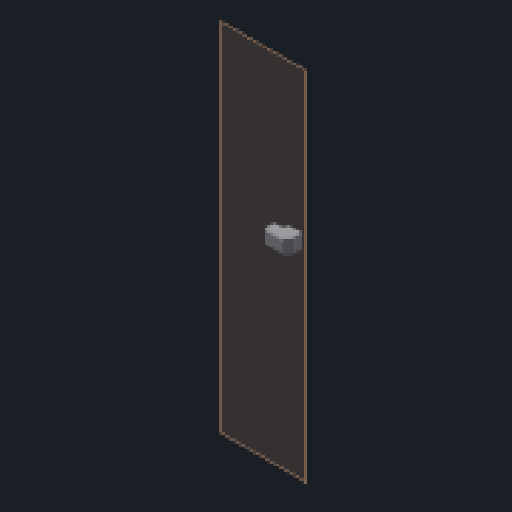
# Autodesk Inventor part: soporte_sensor_puerta
Saved by Autodesk Inventor 2024.3 (Build 283343000, 343)
## iProperties
Created: 2024-08-14
Part Number: soporte_sensor_puerta
Material: Generic
Document SubType Name: Modeling
Designer: Niler
Density: 1 g/cm^3
Appearance: Default
Author: Niler
Autodesk Inventor part; units mm, degrees
ref_plane "YZ Plane" through (0, 0, 0) normal (1, 0, 0) x (0, 1, 0)
ref_plane "XZ Plane" through (0, 0, 0) normal (0, 1, 0) x (-1, 0, 0)
ref_plane "XY Plane" through (0, 0, 0) normal (0, 0, 1) x (1, 0, 0)
ref_plane "Work Plane1" through (0, 0, 0) normal (0, 0, 1) x (1, 0, 0)
sketch "Sketch1" plane through (0, 0, 0) normal (0, 0, 1) x (1, 0, 0)
  line L0 (76.5873, -14.7582) -> (76.5873, 185.2418) projected
  line L1 (76.5873, 107.7418) -> (116.5873, 107.7418)
  line L2 (116.5873, 107.7418) -> (116.5873, 62.7418)
  line L3 (116.5873, 62.7418) -> (76.5873, 62.7418)
  line L4 (76.5873, 62.7418) -> (76.5873, 107.7418)
  point P0 (0, 0)
  point P1 (116.5873, 85.2418)
  point P2 (76.5873, 85.2418)
  point P3 (76.5873, 62.7418)
  dimension "d0" = 45
  dimension "d1" = 40
  constraints: 8 end point, 2 midpoint, 2 parallel, 1 horizontal, 1 horizontal alignment, 1 perpendicular, 1 point on line
  measures "d0" distance of L1.end L2.end
  measures "d1" distance of L2.end L3.end
extrude "Extrusion1" add sketch "Sketch1" along normal blind 45
sketch "Sketch2" plane through (76.5873, 62.7418, 0) normal (-1, 0, 0) x (0, 0, 1)
  line L0 (0, 45) -> (0, 0) projected
  line L1 (0, 0) -> (45, 0) projected
  line L2 (45, 45) -> (45, 0) projected
  line L3 (0, 45) -> (45, 45) projected
  circle A0 centre (29.5, 22.5) radius 9
  point P0 (0, -62.7418)
  point P1 (45, 22.5)
  dimension "d4" = 18
  dimension "d5" = 15.5
  constraints: 1 centre point, 1 horizontal alignment, 1 midpoint
  measures "d4" diameter of A0
  measures "d5" distance from line of A0.centre L2
extrude "Extrusion2" cut sketch "Sketch2" against normal through all contours A0
sketch "Sketch3" plane through (76.5873, 107.7418, 0) normal (0, 1, 0) x (1, 0, 0)
  line L0 (-8, -15) -> (0, -7) projected
  line L1 (-145.0873, -15) -> (-8, -15) projected
  line L2 (-30, -15) -> (-30, -45)
  line L3 (40, 0) -> (0, 0) projected
  line L4 (0, 0) -> (0, -45) projected
  line L5 (40, -45) -> (0, -45) projected
  line L6 (40, 0) -> (40, -45) projected
  line L7 (0, -45) -> (-30, -45)
  point P0 (-76.5873, 0)
  point P1 (0, -7)
  dimension "d8" = 30
  constraints: 5 end point, 1 perpendicular, 1 point on line, 1 vertical
  measures "d8" distance of L4.end L2.end
extrude "Extrusion3" add sketch "Sketch3" against normal up to surface (45 mm away) contours L0 L4 L7 L2 L1
sketch "Sketch4" plane through (46.5873, 107.7418, 15) normal (-1, 0, 0) x (0, 0, 1)
  circle A0 centre (14.5, -22.5) radius 9 projected
  point P0 (-15, -107.7418)
extrude "Extrusion4" cut sketch "Sketch4" against normal through all
chamfer "Chamfer1" distance 15 angle 45 1 edges at (116.5873, 85.2418, 45)
sketch "Sketch5" plane through (101.5873, 62.7418, 45) normal (0.7071068, 0, 0.7071068) x (0.7071068, 0, -0.7071068)
  line L0 (21.2132, 45) -> (0, 45) projected
  line L1 (0, 45) -> (0, 0) projected
  line L2 (0, 0) -> (21.2132, 0) projected
  line L3 (21.2132, 0) -> (21.2132, 13.5139) projected
  ellipse E0 centre (21.9203, 22.5) end of major axis (9.1924, 22.5) minor radius 9 (21.2132, 31.4861) -> (21.2132, 13.5139) ccw projected
  line L4 (21.2132, 31.4861) -> (21.2132, 45) projected
  ellipse E1 centre (21.9203, 22.5) end of major axis (9.1924, 22.5) minor radius 9 (21.2132, 31.4861) -> (21.2132, 13.5139) ccw projected
  line L5 (21.2132, 31.4861) -> (21.2132, 13.5139)
  point P0 (-40.0133, -62.7418)
  constraints: 2 end point, 1 vertical, 2 other
extrude "Extrusion5" add sketch "Sketch5" against normal blind 2
sketch "Sketch6" plane through (116.5873, 62.7418, 0) normal (1, 0, 0) x (0, 0, -1)
  line L0 (-30, 31.4861) -> (-30, 45) projected
  arc A0 (-30, 13.5139) -> (-30, 31.4861) centre (-29.5, 22.5) ccw projected
  line L1 (-30, 0) -> (-30, 13.5139) projected
  line L2 (0, 0) -> (-30, 0) projected
  line L3 (0, 0) -> (0, 45) projected
  line L4 (0, 45) -> (-30, 45) projected
  line L5 (-30, 31.4861) -> (-30, 45) projected
  line L6 (-30, 31.4861) -> (-30, 13.5139)
  point P0 (0, -62.7418)
  constraints: 2 end point, 1 collinear
extrude "Extrusion6" add sketch "Sketch6" against normal blind 2 contours A0 L6
sketch "Sketch7" plane through (0, 0, 0) normal (0, 0, -1) x (-1, 0, 0)
  line L0 (-114.5873, 76.2478) -> (-114.5873, 94.2358) projected
  arc A0 (-114.5873, 76.2478) -> (-114.5873, 94.2358) centre (-114.2589, 85.2418) ccw projected
  point P0 (0, 0)
  point P1 (-46.5873, 94.2418)
  point P2 (-46.5873, 76.2418)
extrude "Extrusion7" cut sketch "Sketch7" against normal blind 50
sketch "Sketch8" plane through (116.5873, 62.7418, 30) normal (0.7071068, 0, 0.7071068) x (0.7071068, 0, -0.7071068)
  ellipse E0 centre (-3.2929, 22.5) end of major axis (9.435, 22.5) minor radius 9 (-2.8284, 31.494) -> (-2.8284, 13.506) ccw projected
  line L0 (-2.8284, 31.494) -> (-2.8284, 13.506) projected
  line L1 (0, 45) -> (-21.2132, 45) projected
  line L2 (-21.2132, 45) -> (-21.2132, 0) projected
  line L3 (-21.2132, 0) -> (0, 0) projected
  line L4 (0, 0) -> (0, 45) projected
  point P0 (-61.2265, -62.7418)
  constraints: 1 other
extrude "Extrusion8" add sketch "Sketch8" against normal blind 2 contours L0 E0 | L4 L3 L2 L1
chamfer "Chamfer2" distance 2 angle 45 6 edges at (109.0873, 107.7418, 37.5) (116.5873, 107.7418, 15) (116.5873, 62.7418, 15) (109.0873, 62.7418, 37.5) (101.5873, 85.2418, 45) (116.5873, 85.2418, 30)
chamfer "Chamfer3" distance 5 angle 45 2 edges at (72.6731, 107.7418, 45) (72.6731, 62.7418, 45)
chamfer "Chamfer4" distance 1 angle 45 5 edges at (46.5873, 107.7418, 27.5) (46.5873, 65.2418, 42.5) (46.5873, 105.2418, 42.5) (46.5873, 85.2418, 45) (46.5873, 62.7418, 27.5)
sketch "Sketch10" plane through (0, 0, 0) normal (0, 0, -1) x (-1, 0, 0)
  line L0 (-114.5873, 62.7418) -> (-116.5873, 64.7418) projected
  line L1 (-76.5873, 62.7418) -> (-114.5873, 62.7418) projected
  line L2 (-76.5873, 107.7418) -> (-76.5873, 62.7418) projected
  line L3 (-114.5873, 107.7418) -> (-76.5873, 107.7418) projected
  line L4 (-116.5873, 105.7418) -> (-114.5873, 107.7418) projected
  line L5 (-116.5873, 64.7418) -> (-116.5873, 105.7418) projected
  arc A0 (-114.5873, 76.2478) -> (-114.5873, 94.2358) centre (-114.2589, 85.2418) ccw projected
  line L6 (-114.5873, 76.2478) -> (-114.5873, 94.2358) projected
  circle A1 centre (-95.5873, 70.7418) radius 1.5
  line L7 (-76.5873, 62.7418) -> (-76.5873, 107.7418) projected
  line L8 (-76.5873, 85.2418) -> (-92.0873, 85.2418)
  circle A2 centre (-95.5873, 99.7418) radius 1.5
  point P0 (0, 0)
  point P1 (-95.5873, 62.7418)
  dimension "d36" = 3
  dimension "d37" = 8
  constraints: 2 centre point, 2 end point, 2 midpoint, 1 horizontal, 1 symmetric about line, 1 vertical alignment, 1 other
  measures "d36" diameter of A1
  measures "d37" distance from line of L1 A1.centre
extrude "Extrusion10" cut sketch "Sketch10" against normal blind 20 contours A1 | A2
sketch "Sketch11" plane through (46.5873, 63.7418, 15) normal (-1, 0, 0) x (0, 0, 1)
  circle A0 centre (14.5, 21.5) radius 8.9 projected
  circle A1 centre (14.5, 21.5) radius 11.7
  line L0 (14.5, 9.2024) -> (3.85, 15.3512)
  line L1 (3.85, 15.3512) -> (3.85, 27.6488)
  line L2 (3.85, 27.6488) -> (14.5, 33.7976)
  line L3 (14.5, 33.7976) -> (25.15, 27.6488)
  line L4 (25.15, 27.6488) -> (25.15, 15.3512)
  line L5 (25.15, 15.3512) -> (14.5, 9.2024)
  point P0 (-15, -63.7418)
  point P1 (25.15, 21.5)
  point P2 (15.6297, 9.8547)
  point P3 (24.0203, 14.699)
  point P4 (25.15, 16.6557)
  point P5 (25.15, 26.3443)
  point P6 (24.0203, 28.301)
  point P7 (15.6297, 33.1453)
  point P8 (13.3703, 33.1453)
  point P9 (4.9797, 28.301)
  point P10 (3.85, 26.3443)
  point P11 (3.85, 16.6557)
  point P12 (4.9797, 14.699)
  point P13 (13.3703, 9.8547)
  dimension "d40" = 23.4
  dimension "d41" = 21.3
  constraints: 12 end point, 2 coincident, 1 centre point, 1 horizontal alignment, 1 midpoint, 13 other
  measures "d40" diameter of A1
  measures "d41" distance between parallel lines of L1 L4
extrude "Extrusion11" cut sketch "Sketch11" against normal blind 8.3 contours L4 A1 L5 L0 L1 L2 L3
sketch "Sketch12" plane through (46.5873, 63.7418, 15) normal (-1, 0, 0) x (0, 0, 1)
  circle A0 centre (14.5, 21.5) radius 11.7 projected
  point P0 (-15, -63.7418)
extrude "Extrusion12" cut sketch "Sketch12" against normal blind 4.1
body "Solid1"
